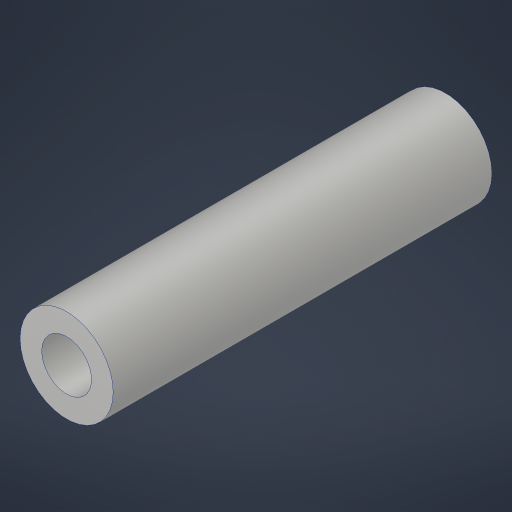
# Autodesk Inventor part: AR-016
Saved by Autodesk Inventor 2023.4 (Build 274418000, 418)
## iProperties
RuleStatus: InUse
Created: 2025-02-15
Part Number: AR-016
Material: Aluminum 6061
Document SubType Name: Modeling
Designer: brand
Density: 2.7 g/cm^3
Appearance: Aluminum - Flat
AfterDocNew0: Open Form 1
Author: brand
Autodesk Inventor part; units mm, degrees
ref_plane "YZ Plane" through (0, 0, 0) normal (1, 0, 0) x (0, 1, 0)
ref_plane "XZ Plane" through (0, 0, 0) normal (0, 1, 0) x (-1, 0, 0)
ref_plane "XY Plane" through (0, 0, 0) normal (0, 0, 1) x (1, 0, 0)
sketch "Sketch1" plane through (0, 0, 0) normal (0, 0, 1) x (1, 0, 0)
  circle A0 centre (0, 0) radius 4.7625
  dimension "d10" = 9.525
  constraints: 2 coincident, 1 centre point
  measures "d10" diameter of A0
extrude "Extrusion1" add sketch "Sketch1" along normal blind 38.7318
hole "Hole1" at (0, 0, 0) direction (0, 0, 1) diameter 5.1054 end through all clearance for "Flat Head Machine Screw (82)" size "#10" standard "Ansi Unified Screw Threads"
equation "\"d10\" = OutsideDiameter"
equation "\"d1\" = StandoffLength"
equation "\"d3\" = HoleDiameter"
equation "\"StandoffLength\" = 38.73183"
equation "\"HoleDiameter\" = 5.1054"
equation "\"OutsideDiameter\" = 9.525"
body "Solid1"
